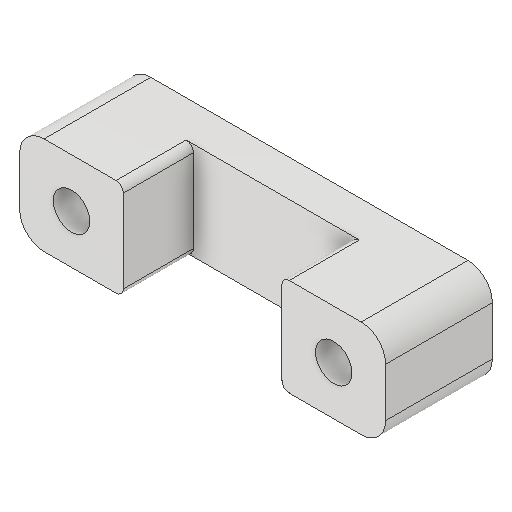
# Autodesk Inventor part: 3DP_PLA_Y_axis_endstop_mount
Saved by Autodesk Inventor 2026.1 (Build 301233000, 233)
## iProperties
Created: 2018-08-01
Part Number: 3DP_PLA_Y_axis_endstop_mount
Material: ABS Plastic
Document SubType Name: Modeling
Designer: Andrzej
Density: 1.06 g/cm^3
Appearance: Smooth - White
Author: Andrzej
Autodesk Inventor part; units mm, degrees
ref_plane "YZ Plane" through (0, 0, 0) normal (1, 0, 0) x (0, 1, 0)
ref_plane "XZ Plane" through (0, 0, 0) normal (0, 1, 0) x (-1, 0, 0)
ref_plane "XY Plane" through (0, 0, 0) normal (0, 0, 1) x (1, 0, 0)
sketch "Sketch1" plane through (0, 0, 0) normal (0, 0, 1) x (1, 0, 0)
  line L0 (-2.4507, 4.6791) -> (10.5493, 4.6791)
  line L1 (10.5493, 4.6791) -> (10.5493, -3.3209)
  line L2 (10.5493, -3.3209) -> (-2.4507, -3.3209)
  line L3 (-2.4507, -3.3209) -> (-2.4507, 4.6791)
  line L4 (-2.4507, 4.6791) -> (-10.9507, 4.6791)
  line L5 (-10.9507, 4.6791) -> (-10.9507, -3.3209)
  line L6 (-10.9507, -3.3209) -> (-2.4507, -3.3209)
  line L7 (10.5493, -3.3209) -> (19.0493, -3.3209)
  line L8 (19.0493, -3.3209) -> (19.0493, 4.6791)
  line L9 (19.0493, 4.6791) -> (10.5493, 4.6791)
  point P0 (0, 0)
  point P1 (-6.7007, 0.6791)
  point P2 (14.7993, 0.6791)
  dimension "d0" = 13
  dimension "d1" = 8
  dimension "d2" = 8.5
  dimension "d3" = 8.5
  dimension "d4" = 30
  dimension "d5" = 4.25
  dimension "d6" = 4
  dimension "d7" = 4
  dimension "d8" = 4.25
  constraints: 20 end point, 5 perpendicular, 2 horizontal, 2 parallel, 2 point on line
  measures "d0" distance of L1.end L2.end
  measures "d1" distance of L2.end L0.start
  measures "d2" distance between parallel lines of L5 L3
  measures "d3" distance between parallel lines of L8 L1
  measures "d4" distance between parallel lines of L8 L5
  measures "d5" distance from line of L5 point (-6.701, 0.679)
  measures "d6" distance from line of L6 point (-6.701, 0.679)
  measures "d7" distance from line of L7 point (14.799, 0.679)
  measures "d8" distance from line of L8 point (14.799, 0.679)
extrude "Extrusion1" add sketch "Sketch1" along normal blind 5.75 contours L3 L6 L5 L4 | L9 L8 L7 L1
extrude "Extrusion2" add sketch "Sketch1" against normal blind 3
hole "Hole1" at (-6.7007, 0.6791, 0) at (14.7993, 0.6791, 0) direction (0, 0, 1) diameter 3 end through all both
fillet "Fillet1" radius 2 2 edges at (-10.9507, -3.3209, 1.375) (-10.9507, 4.6791, 1.375)
fillet "Fillet2" radius 0.6 4 edges at (10.5493, -3.3209, 2.875) (-2.4507, -3.3209, 2.875) (10.5493, 4.6791, 2.875) (-2.4507, 4.6791, 2.875)
equation "\"d3\" = d2"
equation "\"d5\" = 0.5 * d2"
equation "\"d6\" = 0.5 * d1"
equation "\"d7\" = d6"
equation "\"d8\" = d5"
body "Solid1"
